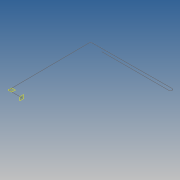
# Autodesk Inventor part: Seil2
Saved by Autodesk Inventor 2015 SP1 (Build 190203100, 203)
## iProperties
Created: 2015-03-05
Part Number: Seil2
Material: Generisch
Document SubType Name: Modeling
Designer: Marc
Density: 1 g/cm^3
Appearance: Vorgabe
Author: Marc
Autodesk Inventor part; units mm, degrees
ref_plane "YZ Plane" through (0, 0, 0) normal (1, 0, 0) x (0, 1, 0)
ref_plane "XZ Plane" through (0, 0, 0) normal (0, 1, 0) x (-1, 0, 0)
ref_plane "XY Plane" through (0, 0, 0) normal (0, 0, 1) x (1, 0, 0)
ref_plane "Arbeitsebene1" through (0, 0, 0) normal (0, 0, 1) x (1, 0, 0)
sketch "Skizze1" plane through (0, 0, 0) normal (0, 0, 1) x (1, 0, 0)
  circle A0 centre (0, 0) radius 10 projected
  arc A1 (-10, 0) -> (0, -10) centre (0, 0) ccw
  line L0 (0, -10) -> (70.0214, -10)
  circle A2 centre (-3.435, 479.9877) radius 10 projected
  arc A3 (-3.435, 489.9877) -> (-13.435, 479.9877) centre (-3.435, 479.9877) ccw
  line L1 (-13.435, 479.9877) -> (-10, 0)
  circle A4 centre (476.5527, 483.4227) radius 10 projected
  line L2 (-3.435, 489.9877) -> (476.4811, 493.4225)
  arc A5 (476.5527, 473.4227) -> (476.4811, 493.4225) centre (476.5527, 483.4227) ccw
  line L3 (476.5527, 473.4227) -> (71.9572, 473.4227)
  point P0 (0, 0)
  constraints: 12 point on circle, 8 end point, 4 tangent, 3 centre point, 3 concentric, 2 horizontal
ref_plane "Arbeitsebene2" through (70.0214, -10, 0) normal (1, 0, 0) x (0, 1, 0)
sketch "Skizze2" plane through (70.0214, -10, 0) normal (1, 0, 0) x (0, 1, 0)
  circle A0 centre (0, 0) radius 1
  point P0 (10, 0)
  dimension "d0" = 2
  constraints: 1 centre point, 1 coincident
  measures "d0" diameter of A0
sweep "Sweeping1" add profiles "Skizze2" path "Skizze1" path curves L0 A1 L1 A3 L2 A5 L3
